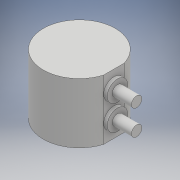
# Autodesk Inventor part: reservoir pump combo pump
Saved by Autodesk Inventor 2018 (Build 220112000, 112)
## iProperties
Created: 2018-06-16
Part Number: reservoir pump combo pump
Material: Generic
Document SubType Name: Modeling
Designer: John Viljoen
Density: 1 g/cm^3
Appearance: Default
Author: John Viljoen
Autodesk Inventor part; units mm, degrees
ref_plane "YZ Plane" through (0, 0, 0) normal (1, 0, 0) x (0, 1, 0)
ref_plane "XZ Plane" through (0, 0, 0) normal (0, 1, 0) x (-1, 0, 0)
ref_plane "XY Plane" through (0, 0, 0) normal (0, 0, 1) x (1, 0, 0)
sketch "Sketch1" plane through (0, 0, 0) normal (0, 0, 1) x (1, 0, 0)
  circle A0 centre (0, 0) radius 30
  dimension "d0" = 60
  constraints: 1 centre point, 1 coincident
  measures "d0" diameter of A0
extrude "Extrusion1" add sketch "Sketch1" along normal blind 50
sketch "Sketch2" plane through (0, 0, 50) normal (0, 0, 1) x (1, 0, 0)
  circle A0 centre (0, 0) radius 30 construction
  line L0 (30, 0) -> (28.75, 0) construction
  line L1 (28.75, 16.5201) -> (34.9612, 16.5201)
  line L2 (34.9612, 16.5201) -> (34.9612, -18.249)
  line L3 (34.9612, -18.249) -> (28.75, -18.249)
  line L4 (28.75, -18.249) -> (28.75, 16.5201)
  dimension "d3" = 1.25
  constraints: 10 end point, 2 horizontal, 2 parallel, 1 horizontal alignment, 1 perpendicular, 1 other
  measures "d3" distance of L0.start L0.end
extrude "Extrusion2" cut sketch "Sketch2" against normal through all
sketch "Sketch3" plane through (28.75, -8.5696, 50) normal (1, 0, 0) x (0, 0, -1)
  line L0 (0, 38.5696) -> (0, -21.4304) construction
  line L1 (0, 8.5696) -> (14, 8.5696) construction
  circle A0 centre (14, 8.5696) radius 8.5
  point P0 (50, 8.5696)
  dimension "d6" = 14
  dimension "d7" = 17
  constraints: 2 end point, 1 centre point, 1 coincident, 1 horizontal, 1 midpoint
  measures "d6" distance of L1.start L1.end
  measures "d7" diameter of A0
extrude "Extrusion3" add sketch "Sketch3" along normal blind 3
sketch "Sketch4" plane through (28.75, -8.5696, 50) normal (1, 0, 0) x (0, 0, -1)
  line L0 (0, 0) -> (0, 17.1391) projected
  line L1 (0, 8.5696) -> (35, 8.5696) construction
  circle A0 centre (35, 8.5696) radius 8.5
  point P0 (50, 8.5696)
  dimension "d10" = 35
  dimension "d11" = 17
  constraints: 2 end point, 1 centre point, 1 coincident, 1 horizontal, 1 midpoint
  measures "d10" distance of L1.start L1.end
  measures "d11" diameter of A0
extrude "Extrusion4" add sketch "Sketch4" along normal blind 3
sketch "Sketch5" plane through (31.75, 0, 36) normal (1, 0, 0) x (0, 0, -1)
  circle A0 centre (0, 0) radius 8.5 projected
  circle A1 centre (0, 0) radius 4.35
  circle A2 centre (21, 0) radius 8.5 projected
  line L0 (12.5, 0) -> (21, 0)
  circle A3 centre (21, 0) radius 4.35
  point P0 (36, 0)
  dimension "d14" = 8.7
  dimension "d15" = 8.7
  constraints: 2 centre point, 2 coincident, 2 end point, 1 horizontal, 1 horizontal alignment, 1 other
  measures "d14" diameter of A1
  measures "d15" diameter of A3
extrude "Extrusion5" add sketch "Sketch5" along normal blind 16 contours A1 | A3
sketch "Sketch6" plane through (28.75, -8.5696, 50) normal (1, 0, 0) x (0, 0, -1)
  line L0 (25, 8.5696) -> (29.25, 8.5696) construction
  line L1 (29.25, 8.5696) -> (29.25, 5.3196) construction
  line L2 (29.25, 5.3196) -> (20.75, 5.3196)
  line L3 (20.75, 5.3196) -> (20.75, 11.8196)
  line L4 (20.75, 11.8196) -> (29.25, 11.8196)
  line L5 (29.25, 11.8196) -> (29.25, 5.3196)
  point P0 (50, 8.5696)
  dimension "d18" = 4.25
  dimension "d19" = 3.25
  dimension "d20" = 8.5
  dimension "d21" = 6.5
  constraints: 12 end point, 2 horizontal, 2 parallel, 2 perpendicular
  measures "d18" distance of L0.start L0.end
  measures "d19" distance of L0.end L1.end
  measures "d20" distance of L3.end L4.end
  measures "d21" distance of L2.end L3.end
extrude "Extrusion6" cut sketch "Sketch6" against normal through all
sketch "Sketch7" plane through (28.75, -8.5696, 50) normal (1, 0, 0) x (0, 0, -1)
  line L0 (29.25, 5.3196) -> (27.1459, 5.3196) projected
  line L1 (29.25, 5.3196) -> (20.75, 5.3196)
  line L2 (20.75, 5.3196) -> (20.75, 11.8196)
  line L3 (20.75, 11.8196) -> (29.25, 11.8196)
  line L4 (29.25, 11.8196) -> (29.25, 5.3196)
  point P0 (50, 8.5696)
  dimension "d24" = 8.5
  dimension "d25" = 6.5
  constraints: 8 end point, 2 parallel, 1 horizontal, 1 perpendicular
  measures "d24" distance of L2.end L3.end
  measures "d25" distance of L1.end L2.end
extrude "Extrusion7" add sketch "Sketch7" against normal blind 55
body "Solid1"
